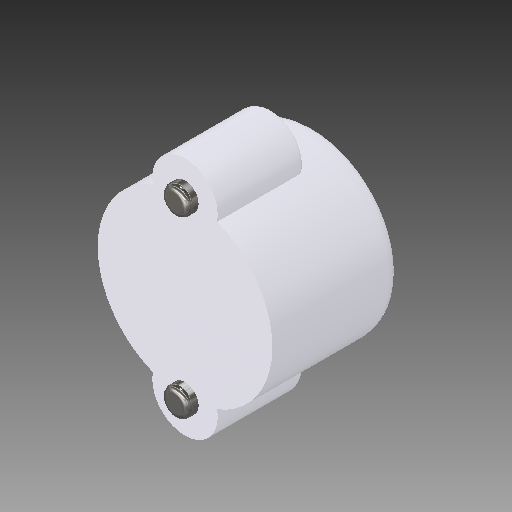
# Autodesk Inventor part: wheel3
Saved by Autodesk Inventor 2017 (Build 210142000, 142)
## iProperties
Created: 2019-12-04
Part Number: wheel3
Material: Generic
Document SubType Name: Modeling
Designer: User
Density: 1 g/cm^3
Appearance: Default
Mass: 2.7213 g
Surface Area: 11.2557 cm^2
Volume: 2.7213 cm^3
Author: User
Autodesk Inventor part; units mm, degrees
ref_plane "YZ Plane" through (0, 0, 0) normal (1, 0, 0) x (0, 1, 0)
ref_plane "XZ Plane" through (0, 0, 0) normal (0, 1, 0) x (-1, 0, 0)
ref_plane "XY Plane" through (0, 0, 0) normal (0, 0, 1) x (1, 0, 0)
sketch "Sketch1" plane through (0, 0, 0) normal (0, 0, 1) x (1, 0, 0)
  circle A0 centre (0, 0) radius 8
  dimension "d0" = 16
  constraints: 1 centre point, 1 coincident
  measures "d0" diameter of A0
extrude "Extrusion1" add sketch "Sketch1" along normal blind 12
sketch "Sketch2" plane through (0, 0, 12) normal (0, 0, 1) x (1, 0, 0)
  circle A0 centre (0, 0) radius 8 projected
  circle A1 centre (0, -8) radius 3
  circle A2 centre (0, 8) radius 3
  dimension "d3" = 6
  dimension "d4" = 6
  constraints: 2 centre point, 2 point on circle
  measures "d3" diameter of A1
  measures "d4" diameter of A2
extrude "Extrusion2" add sketch "Sketch2" against normal blind 8 contours A2 A0 | A0 A2 | A1 A0 | A0 A1
sketch "Sketch4" plane through (0, 0, 0) normal (1, 0, 0) x (0, 1, 0)
  line L0 (0, 0) -> (0, -2)
  arc A0 (-4.899, 0) -> (0, -2) centre (0, 5) ccw
  line L1 (0, 0) -> (-4.899, 0)
  point P0 (-7, 0)
  dimension "d10" = 2
  constraints: 4 end point, 2 point on circle, 1 centre point, 1 horizontal, 1 vertical
  measures "d10" distance of L0.start L0.end
revolve "Revolution1" add sketch "Sketch4" angle 360 about axis through (0, 0, 0) along (0, 0, -1)
fillet "Fillet2" radius 0.5 2 edges at (0, 11, 4) (0, -11, 4)
fillet "Fillet3" radius 1.5 1 edges at (-8, 0, 0)
sketch "Sketch6" plane through (0, 0, 12) normal (0, 0, 1) x (1, 0, 0)
  arc A0 (2.9468, 7.4375) -> (-2.9468, 7.4375) centre (0, 8) ccw projected
  circle A1 centre (0, 8) radius 1.25
  point P0 (0, 0)
  dimension "d16" = 2.5
  constraints: 1 centre point, 1 coincident
  measures "d16" diameter of A1
extrude "Extrusion3" add sketch "Sketch6" along normal blind 1
fillet "Fillet4" radius 0.5 1 edges at (-1.25, 8, 13)
mirror "Mirror1" about plane through (0, 0, 0) normal (0, 1, 0) of "Extrusion3", "Fillet4"
body "Solid1"
